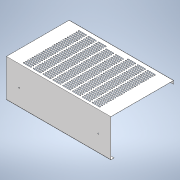
# Autodesk Inventor part: Tapa_superior_superior
Saved by Autodesk Inventor 2021 (Build 250183000, 183)
## iProperties
Created: 2021-04-15
Part Number: Tapa_superior_superior
Material: Genérico
Document SubType Name: Modeling
Designer: Admin
Density: 1 g/cm^3
Appearance: Valor por defecto
Author: Admin
Autodesk Inventor part; units mm, degrees
(part 1 of 2)
ref_plane "YZ Plane" through (0, 0, 0) normal (1, 0, 0) x (0, 1, 0)
ref_plane "XZ Plane" through (0, 0, 0) normal (0, 1, 0) x (-1, 0, 0)
ref_plane "XY Plane" through (0, 0, 0) normal (0, 0, 1) x (1, 0, 0)
sketch "Boceto1" plane through (0, 0, 0) normal (0, 1, 0) x (-1, 0, 0)
  line L0 (0, 0) -> (637.48, 0)
  line L1 (637.48, 0) -> (637.48, -383.48)
  line L2 (637.48, -383.48) -> (0, -383.48)
  line L3 (0, -383.48) -> (0, 0)
  dimension "d0" = 637.48
  dimension "d1" = 383.48
  constraints: 8 end point, 2 parallel, 1 horizontal, 1 perpendicular
  measures "d0" distance of L1.end L2.end
  measures "d1" distance of L0.end L1.end
extrude "Extrusión1" add sketch "Boceto1" along normal blind 0.76
sketch "Boceto2" plane through (0, 0, 0) normal (0, -1, 0) x (1, 0, 0)
  line L0 (0, -383.48) -> (-637.48, -383.48) projected
  line L1 (-637.48, -383.48) -> (-637.48, 0) projected
  line L2 (0, -383.48) -> (-637.48, -383.48)
  line L3 (-637.48, -383.48) -> (-637.48, -382.72)
  line L4 (-637.48, -382.72) -> (0, -382.72)
  line L5 (0, -382.72) -> (0, -383.48)
  point P0 (0, 0)
  dimension "d4" = 0.76
  constraints: 8 end point, 2 parallel, 1 horizontal, 1 perpendicular, 1 point on line
  measures "d4" distance of L2.end L3.end
extrude "Extrusión2" add sketch "Boceto2" along normal blind 19.24
sketch "Boceto4" plane through (0, 0, 0) normal (0, -1, 0) x (1, 0, 0)
  line L0 (-637.48, 0) -> (0, 0) projected
  line L1 (-637.48, -383.48) -> (-637.48, 0) projected
  line L2 (0, 0) -> (-637.48, 0)
  line L3 (-637.48, 0) -> (-637.48, -0.76)
  line L4 (-637.48, -0.76) -> (0, -0.76)
  line L5 (0, -0.76) -> (0, 0)
  dimension "d7" = 0.76
  constraints: 8 end point, 2 parallel, 1 horizontal, 1 perpendicular, 1 point on line
  measures "d7" distance of L3.end L2.end
extrude "Extrusión3" add sketch "Boceto4" along normal blind 227.72
sketch "Boceto5" plane through (0, 0, -0.76) normal (0, 0, -1) x (-1, 0, 0)
  line L0 (0, 0) -> (0, -227.72) projected
  line L1 (637.48, 0) -> (637.48, -227.72) projected
  line L2 (0, -227.72) -> (637.48, -227.72)
  line L3 (637.48, -227.72) -> (637.48, -226.96)
  line L4 (637.48, -226.96) -> (0, -226.96)
  line L5 (0, -226.96) -> (0, -227.72)
  dimension "d10" = 0.76
  constraints: 8 end point, 2 parallel, 1 horizontal, 1 perpendicular, 1 point on line
  measures "d10" distance of L3.end L2.end
extrude "Extrusión4" add sketch "Boceto5" along normal blind 19.24
sketch "Boceto6" plane through (0, 0.76, 0) normal (0, 1, 0) x (1, 0, 0)
  line L0 (-637.48, 0) -> (0, 0) projected
  line L1 (-318.74, 0) -> (-318.74, 383.48)
  line L2 (0, 383.48) -> (-637.48, 383.48) projected
  line L3 (0, 0) -> (0, 383.48) projected
  line L4 (-637.48, 383.48) -> (-637.48, 0) projected
  line L5 (-313.7396, 20.15) -> (-263.7396, 20.15) construction
  line L6 (-310.3896, 23.5) -> (-267.0896, 23.5)
  line L7 (-267.0896, 16.8) -> (-310.3896, 16.8)
  arc A0 (-310.3896, 23.5) -> (-310.3896, 16.8) centre (-310.3896, 20.15) ccw
  arc A1 (-267.0896, 16.8) -> (-267.0896, 23.5) centre (-267.0896, 20.15) ccw
  line L8 (-250.3896, 23.5) -> (-207.0896, 23.5)
  arc A2 (-250.3896, 23.5) -> (-250.3896, 16.8) centre (-250.3896, 20.15) ccw
  line L9 (-207.0896, 16.8) -> (-250.3896, 16.8)
  arc A3 (-207.0896, 16.8) -> (-207.0896, 23.5) centre (-207.0896, 20.15) ccw
  line L10 (-190.3896, 23.5) -> (-147.0896, 23.5)
  arc A4 (-190.3896, 23.5) -> (-190.3896, 16.8) centre (-190.3896, 20.15) ccw
  line L11 (-147.0896, 16.8) -> (-190.3896, 16.8)
  arc A5 (-147.0896, 16.8) -> (-147.0896, 23.5) centre (-147.0896, 20.15) ccw
  line L12 (-130.3896, 23.5) -> (-87.0896, 23.5)
  arc A6 (-130.3896, 23.5) -> (-130.3896, 16.8) centre (-130.3896, 20.15) ccw
  line L13 (-87.0896, 16.8) -> (-130.3896, 16.8)
  arc A7 (-87.0896, 16.8) -> (-87.0896, 23.5) centre (-87.0896, 20.15) ccw
  line L14 (-267.0896, 30.2) -> (-310.3896, 30.2)
  arc A8 (-267.0896, 30.2) -> (-267.0896, 36.9) centre (-267.0896, 33.55) ccw
  line L15 (-310.3896, 36.9) -> (-267.0896, 36.9)
  arc A9 (-310.3896, 36.9) -> (-310.3896, 30.2) centre (-310.3896, 33.55) ccw
  line L16 (-267.0896, 43.6) -> (-310.3896, 43.6)
  arc A10 (-267.0896, 43.6) -> (-267.0896, 50.3) centre (-267.0896, 46.95) ccw
  line L17 (-310.3896, 50.3) -> (-267.0896, 50.3)
  arc A11 (-310.3896, 50.3) -> (-310.3896, 43.6) centre (-310.3896, 46.95) ccw
  line L18 (-267.0896, 57) -> (-310.3896, 57)
  arc A12 (-267.0896, 57) -> (-267.0896, 63.7) centre (-267.0896, 60.35) ccw
  line L19 (-310.3896, 63.7) -> (-267.0896, 63.7)
  arc A13 (-310.3896, 63.7) -> (-310.3896, 57) centre (-310.3896, 60.35) ccw
  line L20 (-267.0896, 70.4) -> (-310.3896, 70.4)
  arc A14 (-267.0896, 70.4) -> (-267.0896, 77.1) centre (-267.0896, 73.75) ccw
  line L21 (-310.3896, 77.1) -> (-267.0896, 77.1)
  arc A15 (-310.3896, 77.1) -> (-310.3896, 70.4) centre (-310.3896, 73.75) ccw
  line L22 (-267.0896, 83.8) -> (-310.3896, 83.8)
  arc A16 (-267.0896, 83.8) -> (-267.0896, 90.5) centre (-267.0896, 87.15) ccw
  line L23 (-310.3896, 90.5) -> (-267.0896, 90.5)
  arc A17 (-310.3896, 90.5) -> (-310.3896, 83.8) centre (-310.3896, 87.15) ccw
  line L24 (-267.0896, 97.2) -> (-310.3896, 97.2)
  arc A18 (-267.0896, 97.2) -> (-267.0896, 103.9) centre (-267.0896, 100.55) ccw
  line L25 (-310.3896, 103.9) -> (-267.0896, 103.9)
  arc A19 (-310.3896, 103.9) -> (-310.3896, 97.2) centre (-310.3896, 100.55) ccw
  line L26 (-267.0896, 110.6) -> (-310.3896, 110.6)
  arc A20 (-267.0896, 110.6) -> (-267.0896, 117.3) centre (-267.0896, 113.95) ccw
  line L27 (-310.3896, 117.3) -> (-267.0896, 117.3)
  arc A21 (-310.3896, 117.3) -> (-310.3896, 110.6) centre (-310.3896, 113.95) ccw
  line L28 (-267.0896, 124) -> (-310.3896, 124)
  arc A22 (-267.0896, 124) -> (-267.0896, 130.7) centre (-267.0896, 127.35) ccw
  line L29 (-310.3896, 130.7) -> (-267.0896, 130.7)
  arc A23 (-310.3896, 130.7) -> (-310.3896, 124) centre (-310.3896, 127.35) ccw
  line L30 (-267.0896, 137.4) -> (-310.3896, 137.4)
  arc A24 (-267.0896, 137.4) -> (-267.0896, 144.1) centre (-267.0896, 140.75) ccw
  line L31 (-310.3896, 144.1) -> (-267.0896, 144.1)
  arc A25 (-310.3896, 144.1) -> (-310.3896, 137.4) centre (-310.3896, 140.75) ccw
  line L32 (-267.0896, 150.8) -> (-310.3896, 150.8)
  arc A26 (-267.0896, 150.8) -> (-267.0896, 157.5) centre (-267.0896, 154.15) ccw
  line L33 (-310.3896, 157.5) -> (-267.0896, 157.5)
  arc A27 (-310.3896, 157.5) -> (-310.3896, 150.8) centre (-310.3896, 154.15) ccw
  line L34 (-267.0896, 164.2) -> (-310.3896, 164.2)
  arc A28 (-267.0896, 164.2) -> (-267.0896, 170.9) centre (-267.0896, 167.55) ccw
  line L35 (-310.3896, 170.9) -> (-267.0896, 170.9)
  arc A29 (-310.3896, 170.9) -> (-310.3896, 164.2) centre (-310.3896, 167.55) ccw
  line L36 (-267.0896, 177.6) -> (-310.3896, 177.6)
  arc A30 (-267.0896, 177.6) -> (-267.0896, 184.3) centre (-267.0896, 180.95) ccw
  line L37 (-310.3896, 184.3) -> (-267.0896, 184.3)
  arc A31 (-310.3896, 184.3) -> (-310.3896, 177.6) centre (-310.3896, 180.95) ccw
  line L38 (-267.0896, 191) -> (-310.3896, 191)
  arc A32 (-267.0896, 191) -> (-267.0896, 197.7) centre (-267.0896, 194.35) ccw
  line L39 (-310.3896, 197.7) -> (-267.0896, 197.7)
  arc A33 (-310.3896, 197.7) -> (-310.3896, 191) centre (-310.3896, 194.35) ccw
  line L40 (-267.0896, 204.4) -> (-310.3896, 204.4)
  arc A34 (-267.0896, 204.4) -> (-267.0896, 211.1) centre (-267.0896, 207.75) ccw
  line L41 (-310.3896, 211.1) -> (-267.0896, 211.1)
  arc A35 (-310.3896, 211.1) -> (-310.3896, 204.4) centre (-310.3896, 207.75) ccw
  line L42 (-267.0896, 217.8) -> (-310.3896, 217.8)
  arc A36 (-267.0896, 217.8) -> (-267.0896, 224.5) centre (-267.0896, 221.15) ccw
  line L43 (-310.3896, 224.5) -> (-267.0896, 224.5)
  arc A37 (-310.3896, 224.5) -> (-310.3896, 217.8) centre (-310.3896, 221.15) ccw
  line L44 (-267.0896, 231.2) -> (-310.3896, 231.2)
  arc A38 (-267.0896, 231.2) -> (-267.0896, 237.9) centre (-267.0896, 234.55) ccw
  line L45 (-310.3896, 237.9) -> (-267.0896, 237.9)
  arc A39 (-310.3896, 237.9) -> (-310.3896, 231.2) centre (-310.3896, 234.55) ccw
  line L46 (-267.0896, 244.6) -> (-310.3896, 244.6)
  arc A40 (-267.0896, 244.6) -> (-267.0896, 251.3) centre (-267.0896, 247.95) ccw
  line L47 (-310.3896, 251.3) -> (-267.0896, 251.3)
  arc A41 (-310.3896, 251.3) -> (-310.3896, 244.6) centre (-310.3896, 247.95) ccw
  line L48 (-267.0896, 258) -> (-310.3896, 258)
  arc A42 (-267.0896, 258) -> (-267.0896, 264.7) centre (-267.0896, 261.35) ccw
  line L49 (-310.3896, 264.7) -> (-267.0896, 264.7)
  arc A43 (-310.3896, 264.7) -> (-310.3896, 258) centre (-310.3896, 261.35) ccw
  line L50 (-267.0896, 271.4) -> (-310.3896, 271.4)
  arc A44 (-267.0896, 271.4) -> (-267.0896, 278.1) centre (-267.0896, 274.75) ccw
  line L51 (-310.3896, 278.1) -> (-267.0896, 278.1)
  arc A45 (-310.3896, 278.1) -> (-310.3896, 271.4) centre (-310.3896, 274.75) ccw
  line L52 (-267.0896, 284.8) -> (-310.3896, 284.8)
  arc A46 (-267.0896, 284.8) -> (-267.0896, 291.5) centre (-267.0896, 288.15) ccw
  line L53 (-310.3896, 291.5) -> (-267.0896, 291.5)
  arc A47 (-310.3896, 291.5) -> (-310.3896, 284.8) centre (-310.3896, 288.15) ccw
  line L54 (-267.0896, 298.2) -> (-310.3896, 298.2)
  arc A48 (-267.0896, 298.2) -> (-267.0896, 304.9) centre (-267.0896, 301.55) ccw
  line L55 (-310.3896, 304.9) -> (-267.0896, 304.9)
  arc A49 (-310.3896, 304.9) -> (-310.3896, 298.2) centre (-310.3896, 301.55) ccw
  line L56 (-267.0896, 311.6) -> (-310.3896, 311.6)
  arc A50 (-267.0896, 311.6) -> (-267.0896, 318.3) centre (-267.0896, 314.95) ccw
  line L57 (-310.3896, 318.3) -> (-267.0896, 318.3)
  arc A51 (-310.3896, 318.3) -> (-310.3896, 311.6) centre (-310.3896, 314.95) ccw
  line L58 (-267.0896, 325) -> (-310.3896, 325)
  arc A52 (-267.0896, 325) -> (-267.0896, 331.7) centre (-267.0896, 328.35) ccw
  line L59 (-310.3896, 331.7) -> (-267.0896, 331.7)
  arc A53 (-310.3896, 331.7) -> (-310.3896, 325) centre (-310.3896, 328.35) ccw
  line L60 (-267.0896, 338.4) -> (-310.3896, 338.4)
  arc A54 (-267.0896, 338.4) -> (-267.0896, 345.1) centre (-267.0896, 341.75) ccw
  line L61 (-310.3896, 345.1) -> (-267.0896, 345.1)
  arc A55 (-310.3896, 345.1) -> (-310.3896, 338.4) centre (-310.3896, 341.75) ccw
  line L62 (-250.3896, 36.9) -> (-207.0896, 36.9)
  arc A56 (-207.0896, 30.2) -> (-207.0896, 36.9) centre (-207.0896, 33.55) ccw
  line L63 (-207.0896, 30.2) -> (-250.3896, 30.2)
  arc A57 (-250.3896, 36.9) -> (-250.3896, 30.2) centre (-250.3896, 33.55) ccw
  arc A58 (-190.3896, 36.9) -> (-190.3896, 30.2) centre (-190.3896, 33.55) ccw
  line L64 (-190.3896, 36.9) -> (-147.0896, 36.9)
  line L65 (-147.0896, 30.2) -> (-190.3896, 30.2)
  arc A59 (-147.0896, 30.2) -> (-147.0896, 36.9) centre (-147.0896, 33.55) ccw
  arc A60 (-130.3896, 36.9) -> (-130.3896, 30.2) centre (-130.3896, 33.55) ccw
  line L66 (-130.3896, 36.9) -> (-87.0896, 36.9)
  line L67 (-87.0896, 30.2) -> (-130.3896, 30.2)
  arc A61 (-87.0896, 30.2) -> (-87.0896, 36.9) centre (-87.0896, 33.55) ccw
  line L68 (-250.3896, 50.3) -> (-207.0896, 50.3)
  arc A62 (-207.0896, 43.6) -> (-207.0896, 50.3) centre (-207.0896, 46.95) ccw
  line L69 (-207.0896, 43.6) -> (-250.3896, 43.6)
  arc A63 (-250.3896, 50.3) -> (-250.3896, 43.6) centre (-250.3896, 46.95) ccw
  arc A64 (-190.3896, 50.3) -> (-190.3896, 43.6) centre (-190.3896, 46.95) ccw
  line L70 (-190.3896, 50.3) -> (-147.0896, 50.3)
  line L71 (-147.0896, 43.6) -> (-190.3896, 43.6)
  arc A65 (-147.0896, 43.6) -> (-147.0896, 50.3) centre (-147.0896, 46.95) ccw
  arc A66 (-130.3896, 50.3) -> (-130.3896, 43.6) centre (-130.3896, 46.95) ccw
  line L72 (-130.3896, 50.3) -> (-87.0896, 50.3)
  line L73 (-87.0896, 43.6) -> (-130.3896, 43.6)
  arc A67 (-87.0896, 43.6) -> (-87.0896, 50.3) centre (-87.0896, 46.95) ccw
  line L74 (-250.3896, 63.7) -> (-207.0896, 63.7)
  arc A68 (-207.0896, 57) -> (-207.0896, 63.7) centre (-207.0896, 60.35) ccw
  line L75 (-207.0896, 57) -> (-250.3896, 57)
  arc A69 (-250.3896, 63.7) -> (-250.3896, 57) centre (-250.3896, 60.35) ccw
  arc A70 (-190.3896, 63.7) -> (-190.3896, 57) centre (-190.3896, 60.35) ccw
  line L76 (-190.3896, 63.7) -> (-147.0896, 63.7)
  line L77 (-147.0896, 57) -> (-190.3896, 57)
  arc A71 (-147.0896, 57) -> (-147.0896, 63.7) centre (-147.0896, 60.35) ccw
  arc A72 (-130.3896, 63.7) -> (-130.3896, 57) centre (-130.3896, 60.35) ccw
  line L78 (-130.3896, 63.7) -> (-87.0896, 63.7)
  line L79 (-87.0896, 57) -> (-130.3896, 57)
  arc A73 (-87.0896, 57) -> (-87.0896, 63.7) centre (-87.0896, 60.35) ccw
  line L80 (-250.3896, 77.1) -> (-207.0896, 77.1)
  arc A74 (-207.0896, 70.4) -> (-207.0896, 77.1) centre (-207.0896, 73.75) ccw
  line L81 (-207.0896, 70.4) -> (-250.3896, 70.4)
  arc A75 (-250.3896, 77.1) -> (-250.3896, 70.4) centre (-250.3896, 73.75) ccw
  arc A76 (-190.3896, 77.1) -> (-190.3896, 70.4) centre (-190.3896, 73.75) ccw
  line L82 (-190.3896, 77.1) -> (-147.0896, 77.1)
  line L83 (-147.0896, 70.4) -> (-190.3896, 70.4)
  arc A77 (-147.0896, 70.4) -> (-147.0896, 77.1) centre (-147.0896, 73.75) ccw
  arc A78 (-130.3896, 77.1) -> (-130.3896, 70.4) centre (-130.3896, 73.75) ccw
  line L84 (-130.3896, 77.1) -> (-87.0896, 77.1)
  line L85 (-87.0896, 70.4) -> (-130.3896, 70.4)
  arc A79 (-87.0896, 70.4) -> (-87.0896, 77.1) centre (-87.0896, 73.75) ccw
  line L86 (-250.3896, 90.5) -> (-207.0896, 90.5)
  arc A80 (-207.0896, 83.8) -> (-207.0896, 90.5) centre (-207.0896, 87.15) ccw
  line L87 (-207.0896, 83.8) -> (-250.3896, 83.8)
  arc A81 (-250.3896, 90.5) -> (-250.3896, 83.8) centre (-250.3896, 87.15) ccw
  arc A82 (-190.3896, 90.5) -> (-190.3896, 83.8) centre (-190.3896, 87.15) ccw
  line L88 (-190.3896, 90.5) -> (-147.0896, 90.5)
  line L89 (-147.0896, 83.8) -> (-190.3896, 83.8)
  arc A83 (-147.0896, 83.8) -> (-147.0896, 90.5) centre (-147.0896, 87.15) ccw
  arc A84 (-130.3896, 90.5) -> (-130.3896, 83.8) centre (-130.3896, 87.15) ccw
  line L90 (-130.3896, 90.5) -> (-87.0896, 90.5)
  line L91 (-87.0896, 83.8) -> (-130.3896, 83.8)
  arc A85 (-87.0896, 83.8) -> (-87.0896, 90.5) centre (-87.0896, 87.15) ccw
  line L92 (-250.3896, 103.9) -> (-207.0896, 103.9)
  arc A86 (-207.0896, 97.2) -> (-207.0896, 103.9) centre (-207.0896, 100.55) ccw
  line L93 (-207.0896, 97.2) -> (-250.3896, 97.2)
  arc A87 (-250.3896, 103.9) -> (-250.3896, 97.2) centre (-250.3896, 100.55) ccw
  arc A88 (-190.3896, 103.9) -> (-190.3896, 97.2) centre (-190.3896, 100.55) ccw
  line L94 (-190.3896, 103.9) -> (-147.0896, 103.9)
  line L95 (-147.0896, 97.2) -> (-190.3896, 97.2)
  arc A89 (-147.0896, 97.2) -> (-147.0896, 103.9) centre (-147.0896, 100.55) ccw
  arc A90 (-130.3896, 103.9) -> (-130.3896, 97.2) centre (-130.3896, 100.55) ccw
  line L96 (-130.3896, 103.9) -> (-87.0896, 103.9)
  line L97 (-87.0896, 97.2) -> (-130.3896, 97.2)
  arc A91 (-87.0896, 97.2) -> (-87.0896, 103.9) centre (-87.0896, 100.55) ccw
  line L98 (-250.3896, 117.3) -> (-207.0896, 117.3)
  arc A92 (-207.0896, 110.6) -> (-207.0896, 117.3) centre (-207.0896, 113.95) ccw
  line L99 (-207.0896, 110.6) -> (-250.3896, 110.6)
  arc A93 (-250.3896, 117.3) -> (-250.3896, 110.6) centre (-250.3896, 113.95) ccw
  arc A94 (-190.3896, 117.3) -> (-190.3896, 110.6) centre (-190.3896, 113.95) ccw
  line L100 (-190.3896, 117.3) -> (-147.0896, 117.3)
  line L101 (-147.0896, 110.6) -> (-190.3896, 110.6)
  arc A95 (-147.0896, 110.6) -> (-147.0896, 117.3) centre (-147.0896, 113.95) ccw
  arc A96 (-130.3896, 117.3) -> (-130.3896, 110.6) centre (-130.3896, 113.95) ccw
  line L102 (-130.3896, 117.3) -> (-87.0896, 117.3)
  line L103 (-87.0896, 110.6) -> (-130.3896, 110.6)
  arc A97 (-87.0896, 110.6) -> (-87.0896, 117.3) centre (-87.0896, 113.95) ccw
  line L104 (-250.3896, 130.7) -> (-207.0896, 130.7)
  arc A98 (-207.0896, 124) -> (-207.0896, 130.7) centre (-207.0896, 127.35) ccw
  line L105 (-207.0896, 124) -> (-250.3896, 124)
  arc A99 (-250.3896, 130.7) -> (-250.3896, 124) centre (-250.3896, 127.35) ccw
  arc A100 (-190.3896, 130.7) -> (-190.3896, 124) centre (-190.3896, 127.35) ccw
  line L106 (-190.3896, 130.7) -> (-147.0896, 130.7)
  line L107 (-147.0896, 124) -> (-190.3896, 124)
  arc A101 (-147.0896, 124) -> (-147.0896, 130.7) centre (-147.0896, 127.35) ccw
  arc A102 (-130.3896, 130.7) -> (-130.3896, 124) centre (-130.3896, 127.35) ccw
  line L108 (-130.3896, 130.7) -> (-87.0896, 130.7)
  line L109 (-87.0896, 124) -> (-130.3896, 124)
  arc A103 (-87.0896, 124) -> (-87.0896, 130.7) centre (-87.0896, 127.35) ccw
  line L110 (-250.3896, 144.1) -> (-207.0896, 144.1)
  arc A104 (-207.0896, 137.4) -> (-207.0896, 144.1) centre (-207.0896, 140.75) ccw
  line L111 (-207.0896, 137.4) -> (-250.3896, 137.4)
  arc A105 (-250.3896, 144.1) -> (-250.3896, 137.4) centre (-250.3896, 140.75) ccw
  arc A106 (-190.3896, 144.1) -> (-190.3896, 137.4) centre (-190.3896, 140.75) ccw
  line L112 (-190.3896, 144.1) -> (-147.0896, 144.1)
  line L113 (-147.0896, 137.4) -> (-190.3896, 137.4)
  arc A107 (-147.0896, 137.4) -> (-147.0896, 144.1) centre (-147.0896, 140.75) ccw
  arc A108 (-130.3896, 144.1) -> (-130.3896, 137.4) centre (-130.3896, 140.75) ccw
  line L114 (-130.3896, 144.1) -> (-87.0896, 144.1)
  line L115 (-87.0896, 137.4) -> (-130.3896, 137.4)
  arc A109 (-87.0896, 137.4) -> (-87.0896, 144.1) centre (-87.0896, 140.75) ccw
  line L116 (-250.3896, 157.5) -> (-207.0896, 157.5)
  arc A110 (-207.0896, 150.8) -> (-207.0896, 157.5) centre (-207.0896, 154.15) ccw
  line L117 (-207.0896, 150.8) -> (-250.3896, 150.8)
  arc A111 (-250.3896, 157.5) -> (-250.3896, 150.8) centre (-250.3896, 154.15) ccw
  arc A112 (-190.3896, 157.5) -> (-190.3896, 150.8) centre (-190.3896, 154.15) ccw
  line L118 (-190.3896, 157.5) -> (-147.0896, 157.5)
  line L119 (-147.0896, 150.8) -> (-190.3896, 150.8)
  arc A113 (-147.0896, 150.8) -> (-147.0896, 157.5) centre (-147.0896, 154.15) ccw
  arc A114 (-130.3896, 157.5) -> (-130.3896, 150.8) centre (-130.3896, 154.15) ccw
  line L120 (-130.3896, 157.5) -> (-87.0896, 157.5)
  line L121 (-87.0896, 150.8) -> (-130.3896, 150.8)
  arc A115 (-87.0896, 150.8) -> (-87.0896, 157.5) centre (-87.0896, 154.15) ccw
  line L122 (-250.3896, 170.9) -> (-207.0896, 170.9)
  arc A116 (-207.0896, 164.2) -> (-207.0896, 170.9) centre (-207.0896, 167.55) ccw
  line L123 (-207.0896, 164.2) -> (-250.3896, 164.2)
  arc A117 (-250.3896, 170.9) -> (-250.3896, 164.2) centre (-250.3896, 167.55) ccw
  arc A118 (-190.3896, 170.9) -> (-190.3896, 164.2) centre (-190.3896, 167.55) ccw
  line L124 (-190.3896, 170.9) -> (-147.0896, 170.9)
  line L125 (-147.0896, 164.2) -> (-190.3896, 164.2)
  arc A119 (-147.0896, 164.2) -> (-147.0896, 170.9) centre (-147.0896, 167.55) ccw
  arc A120 (-130.3896, 170.9) -> (-130.3896, 164.2) centre (-130.3896, 167.55) ccw
  line L126 (-130.3896, 170.9) -> (-87.0896, 170.9)
  line L127 (-87.0896, 164.2) -> (-130.3896, 164.2)
  arc A121 (-87.0896, 164.2) -> (-87.0896, 170.9) centre (-87.0896, 167.55) ccw
  line L128 (-250.3896, 184.3) -> (-207.0896, 184.3)
  arc A122 (-207.0896, 177.6) -> (-207.0896, 184.3) centre (-207.0896, 180.95) ccw
  line L129 (-207.0896, 177.6) -> (-250.3896, 177.6)
  arc A123 (-250.3896, 184.3) -> (-250.3896, 177.6) centre (-250.3896, 180.95) ccw
  arc A124 (-190.3896, 184.3) -> (-190.3896, 177.6) centre (-190.3896, 180.95) ccw
  line L130 (-190.3896, 184.3) -> (-147.0896, 184.3)
  line L131 (-147.0896, 177.6) -> (-190.3896, 177.6)
  arc A125 (-147.0896, 177.6) -> (-147.0896, 184.3) centre (-147.0896, 180.95) ccw
  arc A126 (-130.3896, 184.3) -> (-130.3896, 177.6) centre (-130.3896, 180.95) ccw
  line L132 (-130.3896, 184.3) -> (-87.0896, 184.3)
  line L133 (-87.0896, 177.6) -> (-130.3896, 177.6)
  arc A127 (-87.0896, 177.6) -> (-87.0896, 184.3) centre (-87.0896, 180.95) ccw
  line L134 (-250.3896, 197.7) -> (-207.0896, 197.7)
  arc A128 (-207.0896, 191) -> (-207.0896, 197.7) centre (-207.0896, 194.35) ccw
  line L135 (-207.0896, 191) -> (-250.3896, 191)
  arc A129 (-250.3896, 197.7) -> (-250.3896, 191) centre (-250.3896, 194.35) ccw
  arc A130 (-190.3896, 197.7) -> (-190.3896, 191) centre (-190.3896, 194.35) ccw
  line L136 (-190.3896, 197.7) -> (-147.0896, 197.7)
  line L137 (-147.0896, 191) -> (-190.3896, 191)
  arc A131 (-147.0896, 191) -> (-147.0896, 197.7) centre (-147.0896, 194.35) ccw
  arc A132 (-130.3896, 197.7) -> (-130.3896, 191) centre (-130.3896, 194.35) ccw
  line L138 (-130.3896, 197.7) -> (-87.0896, 197.7)
  line L139 (-87.0896, 191) -> (-130.3896, 191)
  arc A133 (-87.0896, 191) -> (-87.0896, 197.7) centre (-87.0896, 194.35) ccw
  line L140 (-250.3896, 211.1) -> (-207.0896, 211.1)
  arc A134 (-207.0896, 204.4) -> (-207.0896, 211.1) centre (-207.0896, 207.75) ccw
  line L141 (-207.0896, 204.4) -> (-250.3896, 204.4)
  arc A135 (-250.3896, 211.1) -> (-250.3896, 204.4) centre (-250.3896, 207.75) ccw
  arc A136 (-190.3896, 211.1) -> (-190.3896, 204.4) centre (-190.3896, 207.75) ccw
  line L142 (-190.3896, 211.1) -> (-147.0896, 211.1)
  line L143 (-147.0896, 204.4) -> (-190.3896, 204.4)
  arc A137 (-147.0896, 204.4) -> (-147.0896, 211.1) centre (-147.0896, 207.75) ccw
  arc A138 (-130.3896, 211.1) -> (-130.3896, 204.4) centre (-130.3896, 207.75) ccw
  line L144 (-130.3896, 211.1) -> (-87.0896, 211.1)
  line L145 (-87.0896, 204.4) -> (-130.3896, 204.4)
  arc A139 (-87.0896, 204.4) -> (-87.0896, 211.1) centre (-87.0896, 207.75) ccw
  line L146 (-250.3896, 224.5) -> (-207.0896, 224.5)
  arc A140 (-207.0896, 217.8) -> (-207.0896, 224.5) centre (-207.0896, 221.15) ccw
  line L147 (-207.0896, 217.8) -> (-250.3896, 217.8)
  arc A141 (-250.3896, 224.5) -> (-250.3896, 217.8) centre (-250.3896, 221.15) ccw
  arc A142 (-190.3896, 224.5) -> (-190.3896, 217.8) centre (-190.3896, 221.15) ccw
  line L148 (-190.3896, 224.5) -> (-147.0896, 224.5)
  line L149 (-147.0896, 217.8) -> (-190.3896, 217.8)
  arc A143 (-147.0896, 217.8) -> (-147.0896, 224.5) centre (-147.0896, 221.15) ccw
  arc A144 (-130.3896, 224.5) -> (-130.3896, 217.8) centre (-130.3896, 221.15) ccw
  line L150 (-130.3896, 224.5) -> (-87.0896, 224.5)
  line L151 (-87.0896, 217.8) -> (-130.3896, 217.8)
  arc A145 (-87.0896, 217.8) -> (-87.0896, 224.5) centre (-87.0896, 221.15) ccw
  line L152 (-250.3896, 237.9) -> (-207.0896, 237.9)
  arc A146 (-207.0896, 231.2) -> (-207.0896, 237.9) centre (-207.0896, 234.55) ccw
  line L153 (-207.0896, 231.2) -> (-250.3896, 231.2)
  arc A147 (-250.3896, 237.9) -> (-250.3896, 231.2) centre (-250.3896, 234.55) ccw
  arc A148 (-190.3896, 237.9) -> (-190.3896, 231.2) centre (-190.3896, 234.55) ccw
  line L154 (-190.3896, 237.9) -> (-147.0896, 237.9)
  line L155 (-147.0896, 231.2) -> (-190.3896, 231.2)
  arc A149 (-147.0896, 231.2) -> (-147.0896, 237.9) centre (-147.0896, 234.55) ccw
  arc A150 (-130.3896, 237.9) -> (-130.3896, 231.2) centre (-130.3896, 234.55) ccw
  line L156 (-130.3896, 237.9) -> (-87.0896, 237.9)
  line L157 (-87.0896, 231.2) -> (-130.3896, 231.2)
  arc A151 (-87.0896, 231.2) -> (-87.0896, 237.9) centre (-87.0896, 234.55) ccw
  line L158 (-250.3896, 251.3) -> (-207.0896, 251.3)
  arc A152 (-207.0896, 244.6) -> (-207.0896, 251.3) centre (-207.0896, 247.95) ccw
  line L159 (-207.0896, 244.6) -> (-250.3896, 244.6)
  arc A153 (-250.3896, 251.3) -> (-250.3896, 244.6) centre (-250.3896, 247.95) ccw
  arc A154 (-190.3896, 251.3) -> (-190.3896, 244.6) centre (-190.3896, 247.95) ccw
  line L160 (-190.3896, 251.3) -> (-147.0896, 251.3)
  line L161 (-147.0896, 244.6) -> (-190.3896, 244.6)
  arc A155 (-147.0896, 244.6) -> (-147.0896, 251.3) centre (-147.0896, 247.95) ccw
  arc A156 (-130.3896, 251.3) -> (-130.3896, 244.6) centre (-130.3896, 247.95) ccw
  line L162 (-130.3896, 251.3) -> (-87.0896, 251.3)
  line L163 (-87.0896, 244.6) -> (-130.3896, 244.6)
  arc A157 (-87.0896, 244.6) -> (-87.0896, 251.3) centre (-87.0896, 247.95) ccw
  line L164 (-250.3896, 264.7) -> (-207.0896, 264.7)
  arc A158 (-207.0896, 258) -> (-207.0896, 264.7) centre (-207.0896, 261.35) ccw
  line L165 (-207.0896, 258) -> (-250.3896, 258)
  arc A159 (-250.3896, 264.7) -> (-250.3896, 258) centre (-250.3896, 261.35) ccw
  arc A160 (-190.3896, 264.7) -> (-190.3896, 258) centre (-190.3896, 261.35) ccw
  line L166 (-190.3896, 264.7) -> (-147.0896, 264.7)
  line L167 (-147.0896, 258) -> (-190.3896, 258)
  arc A161 (-147.0896, 258) -> (-147.0896, 264.7) centre (-147.0896, 261.35) ccw
  arc A162 (-130.3896, 264.7) -> (-130.3896, 258) centre (-130.3896, 261.35) ccw
  line L168 (-130.3896, 264.7) -> (-87.0896, 264.7)
  line L169 (-87.0896, 258) -> (-130.3896, 258)
  arc A163 (-87.0896, 258) -> (-87.0896, 264.7) centre (-87.0896, 261.35) ccw
  line L170 (-250.3896, 278.1) -> (-207.0896, 278.1)
  arc A164 (-207.0896, 271.4) -> (-207.0896, 278.1) centre (-207.0896, 274.75) ccw
  line L171 (-207.0896, 271.4) -> (-250.3896, 271.4)
  arc A165 (-250.3896, 278.1) -> (-250.3896, 271.4) centre (-250.3896, 274.75) ccw
  arc A166 (-190.3896, 278.1) -> (-190.3896, 271.4) centre (-190.3896, 274.75) ccw
  line L172 (-190.3896, 278.1) -> (-147.0896, 278.1)
  line L173 (-147.0896, 271.4) -> (-190.3896, 271.4)
  arc A167 (-147.0896, 271.4) -> (-147.0896, 278.1) centre (-147.0896, 274.75) ccw
  arc A168 (-130.3896, 278.1) -> (-130.3896, 271.4) centre (-130.3896, 274.75) ccw
  line L174 (-130.3896, 278.1) -> (-87.0896, 278.1)
  line L175 (-87.0896, 271.4) -> (-130.3896, 271.4)
  arc A169 (-87.0896, 271.4) -> (-87.0896, 278.1) centre (-87.0896, 274.75) ccw
  line L176 (-250.3896, 291.5) -> (-207.0896, 291.5)
  arc A170 (-207.0896, 284.8) -> (-207.0896, 291.5) centre (-207.0896, 288.15) ccw
  line L177 (-207.0896, 284.8) -> (-250.3896, 284.8)
  arc A171 (-250.3896, 291.5) -> (-250.3896, 284.8) centre (-250.3896, 288.15) ccw
  arc A172 (-190.3896, 291.5) -> (-190.3896, 284.8) centre (-190.3896, 288.15) ccw
  line L178 (-190.3896, 291.5) -> (-147.0896, 291.5)
  line L179 (-147.0896, 284.8) -> (-190.3896, 284.8)
  arc A173 (-147.0896, 284.8) -> (-147.0896, 291.5) centre (-147.0896, 288.15) ccw
  arc A174 (-130.3896, 291.5) -> (-130.3896, 284.8) centre (-130.3896, 288.15) ccw
  line L180 (-130.3896, 291.5) -> (-87.0896, 291.5)
  line L181 (-87.0896, 284.8) -> (-130.3896, 284.8)
  arc A175 (-87.0896, 284.8) -> (-87.0896, 291.5) centre (-87.0896, 288.15) ccw
  line L182 (-250.3896, 304.9) -> (-207.0896, 304.9)
  arc A176 (-207.0896, 298.2) -> (-207.0896, 304.9) centre (-207.0896, 301.55) ccw
  line L183 (-207.0896, 298.2) -> (-250.3896, 298.2)
  arc A177 (-250.3896, 304.9) -> (-250.3896, 298.2) centre (-250.3896, 301.55) ccw
  arc A178 (-190.3896, 304.9) -> (-190.3896, 298.2) centre (-190.3896, 301.55) ccw
  line L184 (-190.3896, 304.9) -> (-147.0896, 304.9)
  line L185 (-147.0896, 298.2) -> (-190.3896, 298.2)
  arc A179 (-147.0896, 298.2) -> (-147.0896, 304.9) centre (-147.0896, 301.55) ccw
  arc A180 (-130.3896, 304.9) -> (-130.3896, 298.2) centre (-130.3896, 301.55) ccw
  line L186 (-130.3896, 304.9) -> (-87.0896, 304.9)
  line L187 (-87.0896, 298.2) -> (-130.3896, 298.2)
  arc A181 (-87.0896, 298.2) -> (-87.0896, 304.9) centre (-87.0896, 301.55) ccw
  line L188 (-250.3896, 318.3) -> (-207.0896, 318.3)
  arc A182 (-207.0896, 311.6) -> (-207.0896, 318.3) centre (-207.0896, 314.95) ccw
  line L189 (-207.0896, 311.6) -> (-250.3896, 311.6)
  arc A183 (-250.3896, 318.3) -> (-250.3896, 311.6) centre (-250.3896, 314.95) ccw
  arc A184 (-190.3896, 318.3) -> (-190.3896, 311.6) centre (-190.3896, 314.95) ccw
  line L190 (-190.3896, 318.3) -> (-147.0896, 318.3)
  line L191 (-147.0896, 311.6) -> (-190.3896, 311.6)
  arc A185 (-147.0896, 311.6) -> (-147.0896, 318.3) centre (-147.0896, 314.95) ccw
  arc A186 (-130.3896, 318.3) -> (-130.3896, 311.6) centre (-130.3896, 314.95) ccw
  line L192 (-130.3896, 318.3) -> (-87.0896, 318.3)
  line L193 (-87.0896, 311.6) -> (-130.3896, 311.6)
  arc A187 (-87.0896, 311.6) -> (-87.0896, 318.3) centre (-87.0896, 314.95) ccw
  line L194 (-250.3896, 331.7) -> (-207.0896, 331.7)
  arc A188 (-207.0896, 325) -> (-207.0896, 331.7) centre (-207.0896, 328.35) ccw
  line L195 (-207.0896, 325) -> (-250.3896, 325)
  arc A189 (-250.3896, 331.7) -> (-250.3896, 325) centre (-250.3896, 328.35) ccw
  arc A190 (-190.3896, 331.7) -> (-190.3896, 325) centre (-190.3896, 328.35) ccw
  line L196 (-190.3896, 331.7) -> (-147.0896, 331.7)
  line L197 (-147.0896, 325) -> (-190.3896, 325)
  arc A191 (-147.0896, 325) -> (-147.0896, 331.7) centre (-147.0896, 328.35) ccw
  arc A192 (-130.3896, 331.7) -> (-130.3896, 325) centre (-130.3896, 328.35) ccw
  line L198 (-130.3896, 331.7) -> (-87.0896, 331.7)
  line L199 (-87.0896, 325) -> (-130.3896, 325)
  arc A193 (-87.0896, 325) -> (-87.0896, 331.7) centre (-87.0896, 328.35) ccw
  line L200 (-250.3896, 345.1) -> (-207.0896, 345.1)
  arc A194 (-207.0896, 338.4) -> (-207.0896, 345.1) centre (-207.0896, 341.75) ccw
  line L201 (-207.0896, 338.4) -> (-250.3896, 338.4)
  arc A195 (-250.3896, 345.1) -> (-250.3896, 338.4) centre (-250.3896, 341.75) ccw
  arc A196 (-190.3896, 345.1) -> (-190.3896, 338.4) centre (-190.3896, 341.75) ccw
  line L202 (-190.3896, 345.1) -> (-147.0896, 345.1)
  line L203 (-147.0896, 338.4) -> (-190.3896, 338.4)
  arc A197 (-147.0896, 338.4) -> (-147.0896, 345.1) centre (-147.0896, 341.75) ccw
  arc A198 (-130.3896, 345.1) -> (-130.3896, 338.4) centre (-130.3896, 341.75) ccw
  line L204 (-130.3896, 345.1) -> (-87.0896, 345.1)
  line L205 (-87.0896, 338.4) -> (-130.3896, 338.4)
  arc A199 (-87.0896, 338.4) -> (-87.0896, 345.1) centre (-87.0896, 341.75) ccw
  line L206 (-250.3896, 358.5) -> (-207.0896, 358.5)
  arc A200 (-207.0896, 351.8) -> (-207.0896, 358.5) centre (-207.0896, 355.15) ccw
  line L207 (-207.0896, 351.8) -> (-250.3896, 351.8)
  arc A201 (-250.3896, 358.5) -> (-250.3896, 351.8) centre (-250.3896, 355.15) ccw
  arc A202 (-190.3896, 358.5) -> (-190.3896, 351.8) centre (-190.3896, 355.15) ccw
  line L208 (-190.3896, 358.5) -> (-147.0896, 358.5)
  line L209 (-147.0896, 351.8) -> (-190.3896, 351.8)
  arc A203 (-147.0896, 351.8) -> (-147.0896, 358.5) centre (-147.0896, 355.15) ccw
  arc A204 (-130.3896, 358.5) -> (-130.3896, 351.8) centre (-130.3896, 355.15) ccw
  line L210 (-130.3896, 358.5) -> (-87.0896, 358.5)
  line L211 (-87.0896, 351.8) -> (-130.3896, 351.8)
  arc A205 (-87.0896, 351.8) -> (-87.0896, 358.5) centre (-87.0896, 355.15) ccw
  line L212 (-323.7404, 20.15) -> (-373.7404, 20.15) construction
  line L213 (-327.0904, 23.5) -> (-370.3904, 23.5)
  line L214 (-370.3904, 16.8) -> (-327.0904, 16.8)
  arc A206 (-327.0904, 16.8) -> (-327.0904, 23.5) centre (-327.0904, 20.15) ccw
  arc A207 (-370.3904, 23.5) -> (-370.3904, 16.8) centre (-370.3904, 20.15) ccw
  line L215 (-387.0904, 23.5) -> (-430.3904, 23.5)
  arc A208 (-387.0904, 16.8) -> (-387.0904, 23.5) centre (-387.0904, 20.15) ccw
  line L216 (-430.3904, 16.8) -> (-387.0904, 16.8)
  arc A209 (-430.3904, 23.5) -> (-430.3904, 16.8) centre (-430.3904, 20.15) ccw
  line L217 (-447.0904, 23.5) -> (-490.3904, 23.5)
  arc A210 (-447.0904, 16.8) -> (-447.0904, 23.5) centre (-447.0904, 20.15) ccw
  line L218 (-490.3904, 16.8) -> (-447.0904, 16.8)
  arc A211 (-490.3904, 23.5) -> (-490.3904, 16.8) centre (-490.3904, 20.15) ccw
  line L219 (-507.0904, 23.5) -> (-550.3904, 23.5)
  arc A212 (-507.0904, 16.8) -> (-507.0904, 23.5) centre (-507.0904, 20.15) ccw
  line L220 (-550.3904, 16.8) -> (-507.0904, 16.8)
  arc A213 (-550.3904, 23.5) -> (-550.3904, 16.8) centre (-550.3904, 20.15) ccw
  line L221 (-370.3904, 30.2) -> (-327.0904, 30.2)
  arc A214 (-370.3904, 36.9) -> (-370.3904, 30.2) centre (-370.3904, 33.55) ccw
  line L222 (-327.0904, 36.9) -> (-370.3904, 36.9)
  arc A215 (-327.0904, 30.2) -> (-327.0904, 36.9) centre (-327.0904, 33.55) ccw
  line L223 (-370.3904, 43.6) -> (-327.0904, 43.6)
  arc A216 (-370.3904, 50.3) -> (-370.3904, 43.6) centre (-370.3904, 46.95) ccw
  line L224 (-327.0904, 50.3) -> (-370.3904, 50.3)
  arc A217 (-327.0904, 43.6) -> (-327.0904, 50.3) centre (-327.0904, 46.95) ccw
  line L225 (-370.3904, 57) -> (-327.0904, 57)
  arc A218 (-370.3904, 63.7) -> (-370.3904, 57) centre (-370.3904, 60.35) ccw
  line L226 (-327.0904, 63.7) -> (-370.3904, 63.7)
  arc A219 (-327.0904, 57) -> (-327.0904, 63.7) centre (-327.0904, 60.35) ccw
  line L227 (-370.3904, 70.4) -> (-327.0904, 70.4)
  arc A220 (-370.3904, 77.1) -> (-370.3904, 70.4) centre (-370.3904, 73.75) ccw
  line L228 (-327.0904, 77.1) -> (-370.3904, 77.1)
  arc A221 (-327.0904, 70.4) -> (-327.0904, 77.1) centre (-327.0904, 73.75) ccw
  line L229 (-370.3904, 83.8) -> (-327.0904, 83.8)
  arc A222 (-370.3904, 90.5) -> (-370.3904, 83.8) centre (-370.3904, 87.15) ccw
  line L230 (-327.0904, 90.5) -> (-370.3904, 90.5)
  arc A223 (-327.0904, 83.8) -> (-327.0904, 90.5) centre (-327.0904, 87.15) ccw
  line L231 (-370.3904, 97.2) -> (-327.0904, 97.2)
  arc A224 (-370.3904, 103.9) -> (-370.3904, 97.2) centre (-370.3904, 100.55) ccw
  line L232 (-327.0904, 103.9) -> (-370.3904, 103.9)
  arc A225 (-327.0904, 97.2) -> (-327.0904, 103.9) centre (-327.0904, 100.55) ccw
  line L233 (-370.3904, 110.6) -> (-327.0904, 110.6)
  arc A226 (-370.3904, 117.3) -> (-370.3904, 110.6) centre (-370.3904, 113.95) ccw
  line L234 (-327.0904, 117.3) -> (-370.3904, 117.3)
  arc A227 (-327.0904, 110.6) -> (-327.0904, 117.3) centre (-327.0904, 113.95) ccw
  line L235 (-370.3904, 124) -> (-327.0904, 124)
  arc A228 (-370.3904, 130.7) -> (-370.3904, 124) centre (-370.3904, 127.35) ccw
  line L236 (-327.0904, 130.7) -> (-370.3904, 130.7)
  arc A229 (-327.0904, 124) -> (-327.0904, 130.7) centre (-327.0904, 127.35) ccw
  line L237 (-370.3904, 137.4) -> (-327.0904, 137.4)
  arc A230 (-370.3904, 144.1) -> (-370.3904, 137.4) centre (-370.3904, 140.75) ccw
  line L238 (-327.0904, 144.1) -> (-370.3904, 144.1)
  arc A231 (-327.0904, 137.4) -> (-327.0904, 144.1) centre (-327.0904, 140.75) ccw
  line L239 (-370.3904, 150.8) -> (-327.0904, 150.8)
  arc A232 (-370.3904, 157.5) -> (-370.3904, 150.8) centre (-370.3904, 154.15) ccw
  line L240 (-327.0904, 157.5) -> (-370.3904, 157.5)
  arc A233 (-327.0904, 150.8) -> (-327.0904, 157.5) centre (-327.0904, 154.15) ccw
  line L241 (-370.3904, 164.2) -> (-327.0904, 164.2)
  arc A234 (-370.3904, 170.9) -> (-370.3904, 164.2) centre (-370.3904, 167.55) ccw
  line L242 (-327.0904, 170.9) -> (-370.3904, 170.9)
  arc A235 (-327.0904, 164.2) -> (-327.0904, 170.9) centre (-327.0904, 167.55) ccw
  line L243 (-370.3904, 177.6) -> (-327.0904, 177.6)
  arc A236 (-370.3904, 184.3) -> (-370.3904, 177.6) centre (-370.3904, 180.95) ccw
  line L244 (-327.0904, 184.3) -> (-370.3904, 184.3)
  arc A237 (-327.0904, 177.6) -> (-327.0904, 184.3) centre (-327.0904, 180.95) ccw
  line L245 (-370.3904, 191) -> (-327.0904, 191)
  arc A238 (-370.3904, 197.7) -> (-370.3904, 191) centre (-370.3904, 194.35) ccw
  line L246 (-327.0904, 197.7) -> (-370.3904, 197.7)
  arc A239 (-327.0904, 191) -> (-327.0904, 197.7) centre (-327.0904, 194.35) ccw
  line L247 (-370.3904, 204.4) -> (-327.0904, 204.4)
  arc A240 (-370.3904, 211.1) -> (-370.3904, 204.4) centre (-370.3904, 207.75) ccw
  line L248 (-327.0904, 211.1) -> (-370.3904, 211.1)
  arc A241 (-327.0904, 204.4) -> (-327.0904, 211.1) centre (-327.0904, 207.75) ccw
  line L249 (-370.3904, 217.8) -> (-327.0904, 217.8)
  arc A242 (-370.3904, 224.5) -> (-370.3904, 217.8) centre (-370.3904, 221.15) ccw
  line L250 (-327.0904, 224.5) -> (-370.3904, 224.5)
  arc A243 (-327.0904, 217.8) -> (-327.0904, 224.5) centre (-327.0904, 221.15) ccw
  line L251 (-370.3904, 231.2) -> (-327.0904, 231.2)
  arc A244 (-370.3904, 237.9) -> (-370.3904, 231.2) centre (-370.3904, 234.55) ccw
  line L252 (-327.0904, 237.9) -> (-370.3904, 237.9)
  arc A245 (-327.0904, 231.2) -> (-327.0904, 237.9) centre (-327.0904, 234.55) ccw
  line L253 (-370.3904, 244.6) -> (-327.0904, 244.6)
  arc A246 (-370.3904, 251.3) -> (-370.3904, 244.6) centre (-370.3904, 247.95) ccw
  line L254 (-327.0904, 251.3) -> (-370.3904, 251.3)
  arc A247 (-327.0904, 244.6) -> (-327.0904, 251.3) centre (-327.0904, 247.95) ccw
  line L255 (-370.3904, 258) -> (-327.0904, 258)
  arc A248 (-370.3904, 264.7) -> (-370.3904, 258) centre (-370.3904, 261.35) ccw
  line L256 (-327.0904, 264.7) -> (-370.3904, 264.7)
  arc A249 (-327.0904, 258) -> (-327.0904, 264.7) centre (-327.0904, 261.35) ccw
  line L257 (-370.3904, 271.4) -> (-327.0904, 271.4)
  arc A250 (-370.3904, 278.1) -> (-370.3904, 271.4) centre (-370.3904, 274.75) ccw
  line L258 (-327.0904, 278.1) -> (-370.3904, 278.1)
  arc A251 (-327.0904, 271.4) -> (-327.0904, 278.1) centre (-327.0904, 274.75) ccw
  line L259 (-370.3904, 284.8) -> (-327.0904, 284.8)
  arc A252 (-370.3904, 291.5) -> (-370.3904, 284.8) centre (-370.3904, 288.15) ccw
  line L260 (-327.0904, 291.5) -> (-370.3904, 291.5)
  arc A253 (-327.0904, 284.8) -> (-327.0904, 291.5) centre (-327.0904, 288.15) ccw
  line L261 (-370.3904, 298.2) -> (-327.0904, 298.2)
  arc A254 (-370.3904, 304.9) -> (-370.3904, 298.2) centre (-370.3904, 301.55) ccw
  line L262 (-327.0904, 304.9) -> (-370.3904, 304.9)
  arc A255 (-327.0904, 298.2) -> (-327.0904, 304.9) centre (-327.0904, 301.55) ccw
  line L263 (-370.3904, 311.6) -> (-327.0904, 311.6)
  arc A256 (-370.3904, 318.3) -> (-370.3904, 311.6) centre (-370.3904, 314.95) ccw
  line L264 (-327.0904, 318.3) -> (-370.3904, 318.3)
  arc A257 (-327.0904, 311.6) -> (-327.0904, 318.3) centre (-327.0904, 314.95) ccw
  line L265 (-370.3904, 325) -> (-327.0904, 325)
  arc A258 (-370.3904, 331.7) -> (-370.3904, 325) centre (-370.3904, 328.35) ccw
  line L266 (-327.0904, 331.7) -> (-370.3904, 331.7)
  arc A259 (-327.0904, 325) -> (-327.0904, 331.7) centre (-327.0904, 328.35) ccw
  line L267 (-370.3904, 338.4) -> (-327.0904, 338.4)
  arc A260 (-370.3904, 345.1) -> (-370.3904, 338.4) centre (-370.3904, 341.75) ccw
  line L268 (-327.0904, 345.1) -> (-370.3904, 345.1)
  arc A261 (-327.0904, 338.4) -> (-327.0904, 345.1) centre (-327.0904, 341.75) ccw
  line L269 (-387.0904, 36.9) -> (-430.3904, 36.9)
  arc A262 (-430.3904, 36.9) -> (-430.3904, 30.2) centre (-430.3904, 33.55) ccw
  line L270 (-430.3904, 30.2) -> (-387.0904, 30.2)
  arc A263 (-387.0904, 30.2) -> (-387.0904, 36.9) centre (-387.0904, 33.55) ccw
  arc A264 (-447.0904, 30.2) -> (-447.0904, 36.9) centre (-447.0904, 33.55) ccw
  line L271 (-447.0904, 36.9) -> (-490.3904, 36.9)
  line L272 (-490.3904, 30.2) -> (-447.0904, 30.2)
  arc A265 (-490.3904, 36.9) -> (-490.3904, 30.2) centre (-490.3904, 33.55) ccw
  arc A266 (-507.0904, 30.2) -> (-507.0904, 36.9) centre (-507.0904, 33.55) ccw
  line L273 (-507.0904, 36.9) -> (-550.3904, 36.9)
  line L274 (-550.3904, 30.2) -> (-507.0904, 30.2)
  arc A267 (-550.3904, 36.9) -> (-550.3904, 30.2) centre (-550.3904, 33.55) ccw
  line L275 (-387.0904, 50.3) -> (-430.3904, 50.3)
  arc A268 (-430.3904, 50.3) -> (-430.3904, 43.6) centre (-430.3904, 46.95) ccw
  line L276 (-430.3904, 43.6) -> (-387.0904, 43.6)
  arc A269 (-387.0904, 43.6) -> (-387.0904, 50.3) centre (-387.0904, 46.95) ccw
  arc A270 (-447.0904, 43.6) -> (-447.0904, 50.3) centre (-447.0904, 46.95) ccw
  line L277 (-447.0904, 50.3) -> (-490.3904, 50.3)
  line L278 (-490.3904, 43.6) -> (-447.0904, 43.6)
  arc A271 (-490.3904, 50.3) -> (-490.3904, 43.6) centre (-490.3904, 46.95) ccw
  arc A272 (-507.0904, 43.6) -> (-507.0904, 50.3) centre (-507.0904, 46.95) ccw
  line L279 (-507.0904, 50.3) -> (-550.3904, 50.3)
  line L280 (-550.3904, 43.6) -> (-507.0904, 43.6)
  arc A273 (-550.3904, 50.3) -> (-550.3904, 43.6) centre (-550.3904, 46.95) ccw
  line L281 (-387.0904, 63.7) -> (-430.3904, 63.7)
  arc A274 (-430.3904, 63.7) -> (-430.3904, 57) centre (-430.3904, 60.35) ccw
  line L282 (-430.3904, 57) -> (-387.0904, 57)
  arc A275 (-387.0904, 57) -> (-387.0904, 63.7) centre (-387.0904, 60.35) ccw
  arc A276 (-447.0904, 57) -> (-447.0904, 63.7) centre (-447.0904, 60.35) ccw
  line L283 (-447.0904, 63.7) -> (-490.3904, 63.7)
  line L284 (-490.3904, 57) -> (-447.0904, 57)
  arc A277 (-490.3904, 63.7) -> (-490.3904, 57) centre (-490.3904, 60.35) ccw
  arc A278 (-507.0904, 57) -> (-507.0904, 63.7) centre (-507.0904, 60.35) ccw
  line L285 (-507.0904, 63.7) -> (-550.3904, 63.7)
  line L286 (-550.3904, 57) -> (-507.0904, 57)
  arc A279 (-550.3904, 63.7) -> (-550.3904, 57) centre (-550.3904, 60.35) ccw
  line L287 (-387.0904, 77.1) -> (-430.3904, 77.1)
  arc A280 (-430.3904, 77.1) -> (-430.3904, 70.4) centre (-430.3904, 73.75) ccw
  line L288 (-430.3904, 70.4) -> (-387.0904, 70.4)
  arc A281 (-387.0904, 70.4) -> (-387.0904, 77.1) centre (-387.0904, 73.75) ccw
  arc A282 (-447.0904, 70.4) -> (-447.0904, 77.1) centre (-447.0904, 73.75) ccw
  line L289 (-447.0904, 77.1) -> (-490.3904, 77.1)
  line L290 (-490.3904, 70.4) -> (-447.0904, 70.4)
  arc A283 (-490.3904, 77.1) -> (-490.3904, 70.4) centre (-490.3904, 73.75) ccw
  arc A284 (-507.0904, 70.4) -> (-507.0904, 77.1) centre (-507.0904, 73.75) ccw
  line L291 (-507.0904, 77.1) -> (-550.3904, 77.1)
  line L292 (-550.3904, 70.4) -> (-507.0904, 70.4)
  arc A285 (-550.3904, 77.1) -> (-550.3904, 70.4) centre (-550.3904, 73.75) ccw
  line L293 (-387.0904, 90.5) -> (-430.3904, 90.5)
  arc A286 (-430.3904, 90.5) -> (-430.3904, 83.8) centre (-430.3904, 87.15) ccw
  line L294 (-430.3904, 83.8) -> (-387.0904, 83.8)
  arc A287 (-387.0904, 83.8) -> (-387.0904, 90.5) centre (-387.0904, 87.15) ccw
  arc A288 (-447.0904, 83.8) -> (-447.0904, 90.5) centre (-447.0904, 87.15) ccw
  line L295 (-447.0904, 90.5) -> (-490.3904, 90.5)
  line L296 (-490.3904, 83.8) -> (-447.0904, 83.8)
  arc A289 (-490.3904, 90.5) -> (-490.3904, 83.8) centre (-490.3904, 87.15) ccw
  arc A290 (-507.0904, 83.8) -> (-507.0904, 90.5) centre (-507.0904, 87.15) ccw
  line L297 (-507.0904, 90.5) -> (-550.3904, 90.5)
  line L298 (-550.3904, 83.8) -> (-507.0904, 83.8)
  arc A291 (-550.3904, 90.5) -> (-550.3904, 83.8) centre (-550.3904, 87.15) ccw
  line L299 (-387.0904, 103.9) -> (-430.3904, 103.9)
  arc A292 (-430.3904, 103.9) -> (-430.3904, 97.2) centre (-430.3904, 100.55) ccw
  line L300 (-430.3904, 97.2) -> (-387.0904, 97.2)
  arc A293 (-387.0904, 97.2) -> (-387.0904, 103.9) centre (-387.0904, 100.55) ccw
  arc A294 (-447.0904, 97.2) -> (-447.0904, 103.9) centre (-447.0904, 100.55) ccw
  line L301 (-447.0904, 103.9) -> (-490.3904, 103.9)
  line L302 (-490.3904, 97.2) -> (-447.0904, 97.2)
  arc A295 (-490.3904, 103.9) -> (-490.3904, 97.2) centre (-490.3904, 100.55) ccw
  arc A296 (-507.0904, 97.2) -> (-507.0904, 103.9) centre (-507.0904, 100.55) ccw
  line L303 (-507.0904, 103.9) -> (-550.3904, 103.9)
  line L304 (-550.3904, 97.2) -> (-507.0904, 97.2)
  arc A297 (-550.3904, 103.9) -> (-550.3904, 97.2) centre (-550.3904, 100.55) ccw
  line L305 (-387.0904, 117.3) -> (-430.3904, 117.3)
  arc A298 (-430.3904, 117.3) -> (-430.3904, 110.6) centre (-430.3904, 113.95) ccw
  line L306 (-430.3904, 110.6) -> (-387.0904, 110.6)
  arc A299 (-387.0904, 110.6) -> (-387.0904, 117.3) centre (-387.0904, 113.95) ccw
  arc A300 (-447.0904, 110.6) -> (-447.0904, 117.3) centre (-447.0904, 113.95) ccw
  line L307 (-447.0904, 117.3) -> (-490.3904, 117.3)
  line L308 (-490.3904, 110.6) -> (-447.0904, 110.6)
  arc A301 (-490.3904, 117.3) -> (-490.3904, 110.6) centre (-490.3904, 113.95) ccw
  arc A302 (-507.0904, 110.6) -> (-507.0904, 117.3) centre (-507.0904, 113.95) ccw
  line L309 (-507.0904, 117.3) -> (-550.3904, 117.3)
  line L310 (-550.3904, 110.6) -> (-507.0904, 110.6)
  arc A303 (-550.3904, 117.3) -> (-550.3904, 110.6) centre (-550.3904, 113.95) ccw
  line L311 (-387.0904, 130.7) -> (-430.3904, 130.7)
  arc A304 (-430.3904, 130.7) -> (-430.3904, 124) centre (-430.3904, 127.35) ccw
  line L312 (-430.3904, 124) -> (-387.0904, 124)
  arc A305 (-387.0904, 124) -> (-387.0904, 130.7) centre (-387.0904, 127.35) ccw
  arc A306 (-447.0904, 124) -> (-447.0904, 130.7) centre (-447.0904, 127.35) ccw
  line L313 (-447.0904, 130.7) -> (-490.3904, 130.7)
  line L314 (-490.3904, 124) -> (-447.0904, 124)
  arc A307 (-490.3904, 130.7) -> (-490.3904, 124) centre (-490.3904, 127.35) ccw
  arc A308 (-507.0904, 124) -> (-507.0904, 130.7) centre (-507.0904, 127.35) ccw
  line L315 (-507.0904, 130.7) -> (-550.3904, 130.7)
  line L316 (-550.3904, 124) -> (-507.0904, 124)
  arc A309 (-550.3904, 130.7) -> (-550.3904, 124) centre (-550.3904, 127.35) ccw
  line L317 (-387.0904, 144.1) -> (-430.3904, 144.1)
  arc A310 (-430.3904, 144.1) -> (-430.3904, 137.4) centre (-430.3904, 140.75) ccw
  line L318 (-430.3904, 137.4) -> (-387.0904, 137.4)
  arc A311 (-387.0904, 137.4) -> (-387.0904, 144.1) centre (-387.0904, 140.75) ccw
  arc A312 (-447.0904, 137.4) -> (-447.0904, 144.1) centre (-447.0904, 140.75) ccw
  line L319 (-447.0904, 144.1) -> (-490.3904, 144.1)
  line L320 (-490.3904, 137.4) -> (-447.0904, 137.4)
  arc A313 (-490.3904, 144.1) -> (-490.3904, 137.4) centre (-490.3904, 140.75) ccw
  arc A314 (-507.0904, 137.4) -> (-507.0904, 144.1) centre (-507.0904, 140.75) ccw
  line L321 (-507.0904, 144.1) -> (-550.3904, 144.1)
  line L322 (-550.3904, 137.4) -> (-507.0904, 137.4)
  arc A315 (-550.3904, 144.1) -> (-550.3904, 137.4) centre (-550.3904, 140.75) ccw
  line L323 (-387.0904, 157.5) -> (-430.3904, 157.5)
  arc A316 (-430.3904, 157.5) -> (-430.3904, 150.8) centre (-430.3904, 154.15) ccw
  line L324 (-430.3904, 150.8) -> (-387.0904, 150.8)
  arc A317 (-387.0904, 150.8) -> (-387.0904, 157.5) centre (-387.0904, 154.15) ccw
  arc A318 (-447.0904, 150.8) -> (-447.0904, 157.5) centre (-447.0904, 154.15) ccw
  line L325 (-447.0904, 157.5) -> (-490.3904, 157.5)
  line L326 (-490.3904, 150.8) -> (-447.0904, 150.8)
  arc A319 (-490.3904, 157.5) -> (-490.3904, 150.8) centre (-490.3904, 154.15) ccw
  arc A320 (-507.0904, 150.8) -> (-507.0904, 157.5) centre (-507.0904, 154.15) ccw
  line L327 (-507.0904, 157.5) -> (-550.3904, 157.5)
  line L328 (-550.3904, 150.8) -> (-507.0904, 150.8)
  arc A321 (-550.3904, 157.5) -> (-550.3904, 150.8) centre (-550.3904, 154.15) ccw
  line L329 (-387.0904, 170.9) -> (-430.3904, 170.9)
  arc A322 (-430.3904, 170.9) -> (-430.3904, 164.2) centre (-430.3904, 167.55) ccw
  line L330 (-430.3904, 164.2) -> (-387.0904, 164.2)
  arc A323 (-387.0904, 164.2) -> (-387.0904, 170.9) centre (-387.0904, 167.55) ccw
  arc A324 (-447.0904, 164.2) -> (-447.0904, 170.9) centre (-447.0904, 167.55) ccw
  line L331 (-447.0904, 170.9) -> (-490.3904, 170.9)
  line L332 (-490.3904, 164.2) -> (-447.0904, 164.2)
  arc A325 (-490.3904, 170.9) -> (-490.3904, 164.2) centre (-490.3904, 167.55) ccw
  arc A326 (-507.0904, 164.2) -> (-507.0904, 170.9) centre (-507.0904, 167.55) ccw
  line L333 (-507.0904, 170.9) -> (-550.3904, 170.9)
  line L334 (-550.3904, 164.2) -> (-507.0904, 164.2)
  arc A327 (-550.3904, 170.9) -> (-550.3904, 164.2) centre (-550.3904, 167.55) ccw
  line L335 (-387.0904, 184.3) -> (-430.3904, 184.3)
  arc A328 (-430.3904, 184.3) -> (-430.3904, 177.6) centre (-430.3904, 180.95) ccw
  line L336 (-430.3904, 177.6) -> (-387.0904, 177.6)
  arc A329 (-387.0904, 177.6) -> (-387.0904, 184.3) centre (-387.0904, 180.95) ccw
  arc A330 (-447.0904, 177.6) -> (-447.0904, 184.3) centre (-447.0904, 180.95) ccw
  line L337 (-447.0904, 184.3) -> (-490.3904, 184.3)
  line L338 (-490.3904, 177.6) -> (-447.0904, 177.6)
  arc A331 (-490.3904, 184.3) -> (-490.3904, 177.6) centre (-490.3904, 180.95) ccw
  arc A332 (-507.0904, 177.6) -> (-507.0904, 184.3) centre (-507.0904, 180.95) ccw
  line L339 (-507.0904, 184.3) -> (-550.3904, 184.3)
  line L340 (-550.3904, 177.6) -> (-507.0904, 177.6)
  arc A333 (-550.3904, 184.3) -> (-550.3904, 177.6) centre (-550.3904, 180.95) ccw
  line L341 (-387.0904, 197.7) -> (-430.3904, 197.7)
  arc A334 (-430.3904, 197.7) -> (-430.3904, 191) centre (-430.3904, 194.35) ccw
  line L342 (-430.3904, 191) -> (-387.0904, 191)
  arc A335 (-387.0904, 191) -> (-387.0904, 197.7) centre (-387.0904, 194.35) ccw
  arc A336 (-447.0904, 191) -> (-447.0904, 197.7) centre (-447.0904, 194.35) ccw
  line L343 (-447.0904, 197.7) -> (-490.3904, 197.7)
  line L344 (-490.3904, 191) -> (-447.0904, 191)
  arc A337 (-490.3904, 197.7) -> (-490.3904, 191) centre (-490.3904, 194.35) ccw
  arc A338 (-507.0904, 191) -> (-507.0904, 197.7) centre (-507.0904, 194.35) ccw
  line L345 (-507.0904, 197.7) -> (-550.3904, 197.7)
  line L346 (-550.3904, 191) -> (-507.0904, 191)
  arc A339 (-550.3904, 197.7) -> (-550.3904, 191) centre (-550.3904, 194.35) ccw
  line L347 (-387.0904, 211.1) -> (-430.3904, 211.1)
  arc A340 (-430.3904, 211.1) -> (-430.3904, 204.4) centre (-430.3904, 207.75) ccw
  line L348 (-430.3904, 204.4) -> (-387.0904, 204.4)
  arc A341 (-387.0904, 204.4) -> (-387.0904, 211.1) centre (-387.0904, 207.75) ccw
  arc A342 (-447.0904, 204.4) -> (-447.0904, 211.1) centre (-447.0904, 207.75) ccw
  line L349 (-447.0904, 211.1) -> (-490.3904, 211.1)
  line L350 (-490.3904, 204.4) -> (-447.0904, 204.4)
  arc A343 (-490.3904, 211.1) -> (-490.3904, 204.4) centre (-490.3904, 207.75) ccw
  arc A344 (-507.0904, 204.4) -> (-507.0904, 211.1) centre (-507.0904, 207.75) ccw
  line L351 (-507.0904, 211.1) -> (-550.3904, 211.1)
  line L352 (-550.3904, 204.4) -> (-507.0904, 204.4)
  arc A345 (-550.3904, 211.1) -> (-550.3904, 204.4) centre (-550.3904, 207.75) ccw
  line L353 (-387.0904, 224.5) -> (-430.3904, 224.5)
  arc A346 (-430.3904, 224.5) -> (-430.3904, 217.8) centre (-430.3904, 221.15) ccw
  line L354 (-430.3904, 217.8) -> (-387.0904, 217.8)
  arc A347 (-387.0904, 217.8) -> (-387.0904, 224.5) centre (-387.0904, 221.15) ccw
  arc A348 (-447.0904, 217.8) -> (-447.0904, 224.5) centre (-447.0904, 221.15) ccw
  line L355 (-447.0904, 224.5) -> (-490.3904, 224.5)
  line L356 (-490.3904, 217.8) -> (-447.0904, 217.8)
  arc A349 (-490.3904, 224.5) -> (-490.3904, 217.8) centre (-490.3904, 221.15) ccw
  arc A350 (-507.0904, 217.8) -> (-507.0904, 224.5) centre (-507.0904, 221.15) ccw
  line L357 (-507.0904, 224.5) -> (-550.3904, 224.5)
  line L358 (-550.3904, 217.8) -> (-507.0904, 217.8)
  arc A351 (-550.3904, 224.5) -> (-550.3904, 217.8) centre (-550.3904, 221.15) ccw
  line L359 (-387.0904, 237.9) -> (-430.3904, 237.9)